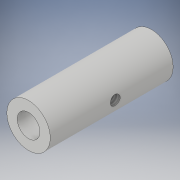
# Autodesk Inventor part: coupler
Saved by Autodesk Inventor 2017 (Build 210142000, 142)
## iProperties
Created: 2016-07-21
Part Number: coupler
Material: Generic
Document SubType Name: Modeling
Designer: Darien Morrow
Density: 1 g/cm^3
Appearance: Default
Author: Darien Morrow
Autodesk Inventor part; units mm, degrees
ref_plane "XZ Plane" through (0, 0, 0) normal (0, 1, 0) x (-1, 0, 0)
ref_plane "XY Plane" through (0, 0, 0) normal (0, 0, 1) x (1, 0, 0)
sketch "Sketch1" plane through (0, 0, 0) normal (0, 0, 1) x (1, 0, 0)
  circle A0 centre (0, 0) radius 4.7625
  dimension "d0" = 9.525
  constraints: 1 centre point, 1 coincident
  measures "d0" diameter of A0
extrude "Extrusion1" add sketch "Sketch1" along normal blind 26.9875
sketch "Sketch2" plane through (0, 0, 26.9875) normal (0, 0, 1) x (1, 0, 0)
  point P0 (0, 0)
  point P1 (0, 0)
  constraints: 1 coincident
hole "Hole1" at (0, 0, 26.9875) direction (0, 0, -1) diameter 5 depth 20.6375 tip angle 118
sketch "Sketch3" plane through (0, 0, 0) normal (0, 0, -1) x (-1, 0, 0)
  circle A0 centre (0, 0) radius 4.7625 projected
  constraints: 1 coincident
hole "Hole2" at (0, 0, 0) direction (0, 0, 1) diameter 2.159 depth 8.8646 tip angle 118
ref_plane "Work Plane1" through (4.7625, 0, 0) normal (1, 0, 0) x (0, 1, 0)
sketch "Sketch4" plane through (4.7625, 0, 0) normal (1, 0, 0) x (0, 1, 0)
  line L0 (-2.5, 26.9875) -> (2.5, 26.9875) projected
  line L1 (0, 26.9875) -> (0, 12.7)
  point P0 (0, 0)
  dimension "d18" = 14.2875
  constraints: 2 end point, 1 coincident, 1 midpoint, 1 vertical
  measures "d18" distance of L1.start L1.end
hole "Hole3" at (4.7625, 0, 12.7) direction (-1, 0, 0) diameter 2.159 depth 3.81 tip angle 118
body "Solid1"
